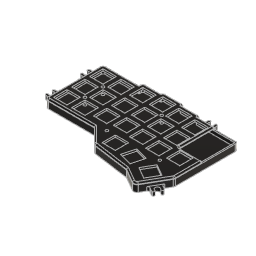
case-tenting-snap (Autodesk Fusion 360 design; units mm, degrees)
Autodesk Fusion 360 part; units mm, degrees
sketch "top_plate" plane through (0, 0, 0) normal (0, 0, 1) x (1, 0, 0)
  arc A0 (37, 57) -> (38, 58) centre (37, 58) ccw
  circle A1 centre (19, 38) radius 1.4
  circle A2 centre (76, 43) radius 1.4
  line L0 (117.5, 20.5) -> (131.5, 20.5)
  arc A3 (114, 24.5) -> (115.5, 23) centre (115.5, 24.5) ccw
  line L1 (95, 60) -> (95, 60)
  line L2 (95, 60) -> (95, 60)
  line L3 (96, 59) -> (112.5, 59)
  arc A4 (66.595, -15.7544) -> (67.4469, -16.1791) centre (67.6556, -14.6937) ccw
  line L4 (123.2697, -29.8066) -> (136.7998, -6.3468)
  arc A5 (106.318, -21.7524) -> (105.7767, -21.566) centre (105.568, -23.0514) ccw
  circle A6 centre (19, 19) radius 1.4
  line L5 (131.5, 20.5) -> (131.5, 6.5)
  line L6 (111.6878, -16.8122) -> (118.6878, -4.6878)
  line L7 (57, 62) -> (57, 62)
  arc A7 (0, 1.5) -> (1.5, 0) centre (1.5, 1.5) ccw
  line L8 (69.5, -13.5) -> (69.5, 0.5)
  line L9 (121.2203, -30.3563) -> (106.318, -21.7524)
  line L10 (118.6878, -4.6878) -> (130.8122, -11.6878)
  line L11 (58, 63) -> (75, 63)
  line L12 (38, 58) -> (38, 60)
  circle A8 centre (61, 0) radius 1.4
  line L13 (1.5, 57) -> (37, 57)
  line L14 (66.595, -15.7544) -> (51.2799, -0.4393)
  line L15 (93.5503, -0.9268) -> (107.0732, -4.5503)
  arc A9 (1.5, 57) -> (0, 55.5) centre (1.5, 55.5) ccw
  arc A10 (95, 60) -> (96, 59) centre (96, 60) ccw
  line L16 (117.5, 6.5) -> (117.5, 20.5)
  line L17 (135.5004, 23) -> (115.5, 23)
  line L18 (114, 24.5) -> (114, 57.5)
  arc A11 (121.2203, -30.3563) -> (123.2697, -29.8066) centre (121.9703, -29.0572) ccw
  arc A12 (136.7998, -6.3468) -> (137.0004, -5.5974) centre (135.5004, -5.5974) ccw
  arc A13 (76, 62) -> (75, 63) centre (75, 62) ccw
  line L19 (105.7767, -21.566) -> (67.4469, -16.1791)
  line L20 (123.8122, -23.8122) -> (111.6878, -16.8122)
  arc A14 (56, 61) -> (57, 62) centre (56, 62) ccw
  line L21 (0, 55.5) -> (0, 1.5)
  arc A15 (58, 63) -> (57, 62) centre (58, 62) ccw
  circle A16 centre (116, 1) radius 1.4
  arc A17 (39, 61) -> (38, 60) centre (39, 60) ccw
  line L22 (76, 62) -> (76, 62)
  line L23 (57, 62) -> (57, 62)
  line L24 (107.0732, -4.5503) -> (103.4497, -18.0732)
  line L25 (103.4497, -18.0732) -> (89.9268, -14.4497)
  line L26 (137.0004, 21.5) -> (137.0004, -5.5974)
  arc A18 (76, 62) -> (77, 61) centre (77, 62) ccw
  line L27 (89.9268, -14.4497) -> (93.5503, -0.9268)
  line L28 (76, 62) -> (76, 62)
  line L29 (1.5, 0) -> (50.2193, 0)
  line L30 (2.5, 40.5) -> (16.5, 40.5)
  line L31 (16.5, 40.5) -> (16.5, 54.5)
  line L32 (2.5, 54.5) -> (2.5, 40.5)
  line L33 (21.5, 2.5) -> (35.5, 2.5)
  line L34 (16.5, 35.5) -> (2.5, 35.5)
  line L35 (35.5, 2.5) -> (35.5, 16.5)
  line L36 (35.5, 21.5) -> (35.5, 35.5)
  line L37 (21.5, 16.5) -> (21.5, 2.5)
  line L38 (16.5, 54.5) -> (2.5, 54.5)
  line L39 (16.5, 21.5) -> (16.5, 35.5)
  line L40 (35.5, 16.5) -> (21.5, 16.5)
  line L41 (2.5, 35.5) -> (2.5, 21.5)
  line L42 (21.5, 21.5) -> (35.5, 21.5)
  line L43 (35.5, 35.5) -> (21.5, 35.5)
  line L44 (69.5, 0.5) -> (83.5, 0.5)
  line L45 (2.5, 21.5) -> (16.5, 21.5)
  line L46 (111.5, 42.5) -> (97.5, 42.5)
  line L47 (59.5, 8.5) -> (59.5, 22.5)
  line L48 (111.5, 37.5) -> (111.5, 23.5)
  line L49 (73.5, 46.5) -> (59.5, 46.5)
  line L50 (73.5, 41.5) -> (73.5, 27.5)
  line L51 (73.5, 22.5) -> (73.5, 8.5)
  line L52 (97.5, 18.5) -> (111.5, 18.5)
  line L53 (92.5, 39.5) -> (78.5, 39.5)
  line L54 (40.5, 20.5) -> (40.5, 6.5)
  line L55 (59.5, 27.5) -> (59.5, 41.5)
  line L56 (111.5, 4.5) -> (97.5, 4.5)
  line L57 (54.5, 44.5) -> (54.5, 58.5)
  line L58 (54.5, 20.5) -> (40.5, 20.5)
  line L59 (16.5, 2.5) -> (16.5, 16.5)
  line L60 (40.5, 39.5) -> (40.5, 25.5)
  line L61 (21.5, 40.5) -> (35.5, 40.5)
  line L62 (97.5, 56.5) -> (111.5, 56.5)
  line L63 (59.5, 60.5) -> (73.5, 60.5)
  line L64 (40.5, 44.5) -> (54.5, 44.5)
  line L65 (111.5, 56.5) -> (111.5, 42.5)
  line L66 (40.5, 25.5) -> (54.5, 25.5)
  line L67 (35.5, 40.5) -> (35.5, 54.5)
  arc A19 (95, 60) -> (94, 61) centre (94, 60) ccw
  line L68 (97.5, 23.5) -> (97.5, 37.5)
  line L69 (35.5, 54.5) -> (21.5, 54.5)
  line L70 (78.5, 39.5) -> (78.5, 25.5)
  line L71 (59.5, 22.5) -> (73.5, 22.5)
  line L72 (92.5, 44.5) -> (92.5, 58.5)
  line L73 (111.5, 23.5) -> (97.5, 23.5)
  line L74 (92.5, 25.5) -> (92.5, 39.5)
  line L75 (131.5, 6.5) -> (117.5, 6.5)
  line L76 (97.5, 4.5) -> (97.5, 18.5)
  line L77 (54.5, 58.5) -> (40.5, 58.5)
  line L78 (83.5, 0.5) -> (83.5, -13.5)
  line L79 (73.5, 8.5) -> (59.5, 8.5)
  line L80 (111.5, 18.5) -> (111.5, 4.5)
  line L81 (21.5, 35.5) -> (21.5, 21.5)
  line L82 (92.5, 6.5) -> (92.5, 20.5)
  line L83 (16.5, 16.5) -> (2.5, 16.5)
  line L84 (59.5, 41.5) -> (73.5, 41.5)
  line L85 (78.5, 6.5) -> (92.5, 6.5)
  line L86 (40.5, 58.5) -> (40.5, 44.5)
  line L87 (92.5, 20.5) -> (78.5, 20.5)
  line L88 (54.5, 25.5) -> (54.5, 39.5)
  line L89 (2.5, 16.5) -> (2.5, 2.5)
  line L90 (73.5, 27.5) -> (59.5, 27.5)
  line L91 (78.5, 25.5) -> (92.5, 25.5)
  line L92 (54.5, 6.5) -> (54.5, 20.5)
  line L93 (92.5, 58.5) -> (78.5, 58.5)
  arc A20 (137.0004, 21.5) -> (135.5004, 23) centre (135.5004, 21.5) ccw
  line L94 (130.8122, -11.6878) -> (123.8122, -23.8122)
  line L95 (39, 61) -> (56, 61)
  line L96 (77, 61) -> (94, 61)
  line L97 (40.5, 6.5) -> (54.5, 6.5)
  arc A21 (114, 57.5) -> (112.5, 59) centre (112.5, 57.5) ccw
  line L98 (97.5, 42.5) -> (97.5, 56.5)
  line L99 (78.5, 44.5) -> (92.5, 44.5)
  line L100 (21.5, 54.5) -> (21.5, 40.5)
  line L101 (73.5, 60.5) -> (73.5, 46.5)
  line L102 (59.5, 46.5) -> (59.5, 60.5)
  line L103 (54.5, 39.5) -> (40.5, 39.5)
  line L104 (78.5, 58.5) -> (78.5, 44.5)
  arc A22 (51.2799, -0.4393) -> (50.2193, 0) centre (50.2193, -1.5) ccw
  line L105 (97.5, 37.5) -> (111.5, 37.5)
  line L106 (83.5, -13.5) -> (69.5, -13.5)
  line L107 (2.5, 2.5) -> (16.5, 2.5)
  line L108 (78.5, 20.5) -> (78.5, 6.5)
  line L109 (77.8284, 63) -> (94, 63)
  arc A23 (96.8284, 61) -> (94, 63) centre (94, 60) ccw
  line L110 (96.8284, 61) -> (112.5, 61)
  line L111 (139.0004, 21.5) -> (139.0004, -5.5974)
  arc A24 (138.5323, -7.346) -> (139.0004, -5.5974) centre (135.5004, -5.5974) ccw
  line L112 (125.0022, -30.8058) -> (138.5323, -7.346)
  arc A25 (120.2203, -32.0883) -> (125.0022, -30.8058) centre (121.9703, -29.0572) ccw
  line L113 (120.2203, -32.0883) -> (105.4021, -23.5331)
  line L114 (105.4021, -23.5331) -> (67.1685, -18.1597)
  arc A26 (65.1808, -17.1686) -> (67.1685, -18.1597) centre (67.6556, -14.6937) ccw
  line L115 (65.1808, -17.1686) -> (50.0122, -2)
  line L116 (1.5, -2) -> (50.0122, -2)
  arc A27 (-2, 1.5) -> (1.5, -2) centre (1.5, 1.5) ccw
  line L117 (-2, 55.5) -> (-2, 1.5)
  arc A28 (1.5, 59) -> (-2, 55.5) centre (1.5, 55.5) ccw
  line L118 (1.5, 59) -> (36, 59)
  line L119 (36, 59) -> (36, 60)
  arc A29 (39, 63) -> (36, 60) centre (39, 60) ccw
  line L120 (39, 63) -> (55.1716, 63)
  arc A30 (58, 65) -> (55.1716, 63) centre (58, 62) ccw
  line L121 (58, 65) -> (75, 65)
  arc A31 (77.8284, 63) -> (75, 65) centre (75, 62) ccw
  line L122 (114, 57.5) -> (114, 59.5)
  line L123 (135.5004, 23) -> (137.5004, 23)
  arc A32 (114, 59.5) -> (112.5, 61) centre (112.5, 59.5) ccw
  arc A33 (139.0004, 21.5) -> (137.5004, 23) centre (137.5004, 21.5) ccw
  dimension "d10" = 1.5
  dimension "d11" = 1.5
  constraint tangent A21 L122
  constraint perpendicular L110 L122
  constraint parallel L96 L109
  constraint concentric A19 A23
  constraint parallel L3 L110
  constraint parallel L26 L111
  constraint concentric A12 A24
  constraint parallel L4 L112
  constraint concentric A11 A25
  constraint parallel L9 L113
  constraint parallel L19 L114
  constraint concentric A4 A26
  constraint parallel L14 L115
  constraint parallel L29 L116
  constraint concentric A7 A27
  constraint parallel L21 L117
  constraint concentric A9 A28
  constraint parallel L13 L118
  constraint parallel L12 L119
  constraint concentric A17 A29
  constraint parallel L95 L120
  constraint concentric A15 A30
  constraint parallel L11 L121
  constraint concentric A13 A31
  constraint tangent L109 A23
  constraint tangent A29 L120
  constraint tangent L111 A24
  constraint tangent A24 L112
  constraint tangent L112 A25
  constraint tangent A25 L113
  constraint tangent L114 A26
  constraint tangent A26 L115
  constraint tangent L116 A27
  constraint tangent A27 L117
  constraint tangent L117 A28
  constraint tangent A28 L118
  constraint tangent L119 A29
  constraint tangent A30 L121
  constraint tangent L121 A31
  constraint tangent A20 L123
  constraint perpendicular L111 L123
  constraint tangent L110 A32
  constraint tangent L122 A32
  constraint tangent L123 A33
  constraint tangent L111 A33
  measures "d10" radius of A32
  measures "d11" radius of A33
extrude "Extrude4" add sketch "top_plate" along normal blind 2 makes body 1
fillet "Fillet1" radius 1.5 27 edges at (18.75, 59, 2) (-0.9749, 57.9749, 2) (-2, 28.5, 2) (-0.9749, -0.9749, 2) (25.7561, -2, 2) (57.5965, -9.5843, 2) (66.0939, -17.826, 2) (86.2853, -20.8464, 2) (112.8112, -27.8107, 2) (122.8769, -32.4378, 2) (131.7673, -19.0759, 2) (138.8814, -6.5025, 2) (139.0004, 7.9513, 2) (138.5611, 22.5607, 2) (126.5002, 23, 2) (114.4393, 23.4393, 2) (114, 42, 2) (113.5607, 60.5607, 2) (104.6642, 61, 2) (95.7321, 62.4495, 2) (85.9142, 63, 2) (76.7321, 64.4495, 2) (66.5, 65, 2) (56.2679, 64.4495, 2) (47.0858, 63, 2) (36.8787, 62.1213, 2) (36, 59.5, 2) on bodies 1
sketch "bottom_plate" plane through (0, 0, 0) normal (0, 0, 1) x (1, 0, 0) in component "case-bottom"
  circle A0 centre (19, 38) radius 1.4
  circle A1 centre (61, 0) radius 1.4
  circle A2 centre (116, 1) radius 1.4
  arc A3 (56, 61) -> (57, 62) centre (56, 62) ccw
  circle A4 centre (76, 43) radius 1.4
  line L0 (121.2203, -30.3563) -> (106.318, -21.7524)
  line L1 (76, 62) -> (76, 62)
  line L2 (57, 62) -> (57, 62)
  line L3 (105.7767, -21.566) -> (67.4469, -16.1791)
  arc A5 (121.2203, -30.3563) -> (123.2697, -29.8066) centre (121.9703, -29.0572) ccw
  arc A6 (136.7994, -6.3479) -> (137, -5.5984) centre (135.5, -5.5984) ccw
  arc A7 (106.318, -21.7524) -> (105.7767, -21.566) centre (105.568, -23.0514) ccw
  arc A8 (76, 62) -> (75, 63) centre (75, 62) ccw
  line L4 (58, 63) -> (75, 63)
  arc A9 (95, 60) -> (96, 59) centre (96, 60) ccw
  arc A10 (0, 1.5) -> (1.5, 0) centre (1.5, 1.5) ccw
  arc A11 (51.2799, -0.4393) -> (50.2193, 0) centre (50.2193, -1.5) ccw
  line L5 (123.2697, -29.8066) -> (136.7994, -6.3479)
  arc A12 (37, 57) -> (38, 58) centre (37, 58) ccw
  arc A13 (66.595, -15.7544) -> (67.4469, -16.1791) centre (67.6556, -14.6937) ccw
  line L6 (1.5, 0) -> (50.2193, 0)
  line L7 (38, 58) -> (38, 60)
  line L8 (76, 62) -> (76, 62)
  line L9 (39, 61) -> (56, 61)
  arc A14 (39, 61) -> (38, 60) centre (39, 60) ccw
  line L10 (95, 60) -> (95, 60)
  line L11 (95, 60) -> (95, 60)
  line L12 (66.595, -15.7544) -> (51.2799, -0.4393)
  line L13 (0, 55.5) -> (0, 1.5)
  line L14 (1.5, 57) -> (37, 57)
  arc A15 (1.5, 57) -> (0, 55.5) centre (1.5, 55.5) ccw
  line L15 (77, 61) -> (94, 61)
  line L16 (57, 62) -> (57, 62)
  arc A16 (58, 63) -> (57, 62) centre (58, 62) ccw
  circle A17 centre (19, 19) radius 1.4
  line L17 (137, 57.5) -> (137, -5.5984)
  arc A18 (137, 57.5) -> (135.5, 59) centre (135.5, 57.5) ccw
  arc A19 (76, 62) -> (77, 61) centre (77, 62) ccw
  line L18 (95, 60) -> (95, 60)
  arc A20 (95, 60) -> (94, 61) centre (94, 60) ccw
  line L19 (96, 59) -> (135.5, 59)
  line L20 (96.8284, 61) -> (98, 61)
  arc A21 (139, 57.5) -> (135.5, 61) centre (135.5, 57.5) ccw
  line L21 (139, 57.5) -> (139, -5.5984)
  arc A22 (138.5319, -7.3471) -> (139, -5.5984) centre (135.5, -5.5984) ccw
  line L22 (135.2589, -13.0219) -> (138.5319, -7.3471)
  arc A23 (120.2203, -32.0883) -> (125.0022, -30.8059) centre (121.9703, -29.0572) ccw
  line L23 (120.2203, -32.0883) -> (105.4021, -23.5331)
  line L24 (105.4021, -23.5331) -> (67.1685, -18.1597)
  arc A24 (65.1808, -17.1686) -> (67.1685, -18.1597) centre (67.6556, -14.6937) ccw
  line L25 (65.1808, -17.1686) -> (50.0122, -2)
  line L26 (1.5, -2) -> (50.0122, -2)
  arc A25 (-2, 1.5) -> (1.5, -2) centre (1.5, 1.5) ccw
  line L27 (-2, 40.021) -> (-2, 17)
  arc A26 (1.5, 59) -> (-2, 55.5) centre (1.5, 55.5) ccw
  line L28 (1.5, 59) -> (36, 59)
  line L29 (36, 59) -> (36, 60)
  arc A27 (39, 63) -> (36, 60) centre (39, 60) ccw
  line L30 (39, 63) -> (55.1716, 63)
  arc A28 (58, 65) -> (55.1716, 63) centre (58, 62) ccw
  line L31 (58, 65) -> (75, 65)
  arc A29 (77.8284, 63) -> (75, 65) centre (75, 62) ccw
  line L32 (77.8284, 63) -> (94, 63)
  arc A30 (96.8284, 61) -> (94, 63) centre (94, 60) ccw
  arc A31 (95.5, 60) -> (96, 59.5) centre (96, 60) ccw
  line L33 (96, 59.5) -> (135.5, 59.5)
  arc A32 (137.5, 57.5) -> (135.5, 59.5) centre (135.5, 57.5) ccw
  line L34 (137.5, 57.5) -> (137.5, -5.5984)
  arc A33 (137.2325, -6.5977) -> (137.5, -5.5984) centre (135.5, -5.5984) ccw
  line L35 (123.7028, -30.0564) -> (137.2325, -6.5977)
  arc A34 (120.9703, -30.7893) -> (123.7028, -30.0564) centre (121.9703, -29.0572) ccw
  line L36 (120.9703, -30.7893) -> (106.068, -22.1854)
  arc A35 (106.068, -22.1854) -> (105.7071, -22.0612) centre (105.568, -23.0514) ccw
  line L37 (105.7071, -22.0612) -> (67.3773, -16.6743)
  arc A36 (66.2414, -16.1079) -> (67.3773, -16.6743) centre (67.6556, -14.6937) ccw
  line L38 (66.2414, -16.1079) -> (50.9264, -0.7929)
  arc A37 (50.9264, -0.7929) -> (50.2193, -0.5) centre (50.2193, -1.5) ccw
  line L39 (1.5, -0.5) -> (50.2193, -0.5)
  arc A38 (-0.5, 1.5) -> (1.5, -0.5) centre (1.5, 1.5) ccw
  line L40 (-0.5, 55.5) -> (-0.5, 1.5)
  arc A39 (1.5, 57.5) -> (-0.5, 55.5) centre (1.5, 55.5) ccw
  line L41 (1.5, 57.5) -> (37, 57.5)
  arc A40 (37, 57.5) -> (37.5, 58) centre (37, 58) ccw
  line L42 (37.5, 58) -> (37.5, 60)
  arc A41 (39, 61.5) -> (37.5, 60) centre (39, 60) ccw
  line L43 (39, 61.5) -> (56, 61.5)
  arc A42 (56, 61.5) -> (56.5, 62) centre (56, 62) ccw
  arc A43 (58, 63.5) -> (56.5, 62) centre (58, 62) ccw
  line L44 (58, 63.5) -> (75, 63.5)
  arc A44 (76.5, 62) -> (75, 63.5) centre (75, 62) ccw
  arc A45 (76.5, 62) -> (77, 61.5) centre (77, 62) ccw
  line L45 (77, 61.5) -> (94, 61.5)
  arc A46 (95.5, 60) -> (94, 61.5) centre (94, 60) ccw
  line L46 (1.5, 57) -> (1.5, 47) construction
  line L47 (1.5, 0) -> (1.5, 10) construction
  line L48 (1.5, 47) -> (-7.1381, 47) construction
  line L49 (1.5, 10) -> (-7, 10) construction
  circle A47 centre (-7, 10) radius 5 construction
  line L50 (-7, 10) -> (-7, 15) construction
  line L51 (-7, 10) -> (-7, 5) construction
  line L52 (-7, 15) -> (-4, 15)
  line L53 (-7, 5) -> (-4, 5)
  circle A48 centre (-7, 10) radius 2.6
  arc A49 (-7, 15) -> (-9.1131, 14.5315) centre (-7, 10) ccw
  line L54 (-7, 10) -> (-7, 15) construction
  line L55 (-7, 10) -> (-9.1131, 14.5315) construction
  arc A50 (-9.1131, 5.4685) -> (-7, 5) centre (-7, 10) ccw
  line L56 (-7, 10) -> (-9.1131, 5.4685) construction
  line L57 (-7, 10) -> (-7, 5) construction
  line L58 (-9.1131, 14.5315) -> (-8.0988, 12.3564) construction
  line L59 (-9.1131, 5.4685) -> (-8.0988, 7.6436) construction
  arc A51 (-9.1131, 14.5315) -> (-8.0988, 12.3564) centre (-8.6059, 13.444) ccw
  line L60 (-8.6059, 13.444) -> (-9.1131, 14.5315) construction
  line L61 (-8.6059, 13.444) -> (-8.0988, 12.3564) construction
  arc A52 (-8.0988, 7.6436) -> (-9.1131, 5.4685) centre (-8.6059, 6.556) ccw
  line L62 (-8.6059, 6.556) -> (-8.0988, 7.6436) construction
  line L63 (-8.6059, 6.556) -> (-9.1131, 5.4685) construction
  arc A53 (-8.2429, 44.7163) -> (-9.3647, 42.5946) centre (-8.8038, 43.6555) ccw
  arc A54 (-9.1407, 51.5463) -> (-8.1264, 49.3712) centre (-8.6335, 50.4587) ccw
  line L64 (-7.0276, 47.0148) -> (-7.2777, 42.021) construction
  arc A55 (-9.3647, 42.5946) -> (-7.2777, 42.021) centre (-7.0276, 47.0148) ccw
  line L65 (-8.6335, 50.4587) -> (-8.1264, 49.3712) construction
  line L66 (-7.1381, 47) -> (-7.2777, 42.021) construction
  line L67 (-7.1381, 47) -> (-7.0276, 52.0148) construction
  line L68 (-7.0276, 47.0148) -> (-7.0276, 52.0148) construction
  line L69 (-7.0276, 47.0148) -> (-9.3647, 42.5946) construction
  circle A56 centre (-7.0276, 47.0148) radius 2.6
  line L70 (-8.6335, 50.4587) -> (-9.1407, 51.5463) construction
  arc A57 (-7.0276, 52.0148) -> (-9.1407, 51.5463) centre (-7.0276, 47.0148) ccw
  line L71 (-9.1407, 51.5463) -> (-8.1264, 49.3712) construction
  line L72 (-9.3647, 42.5946) -> (-8.2429, 44.7163) construction
  line L73 (-7.0276, 47.0148) -> (-9.1407, 51.5463) construction
  line L74 (-8.8038, 43.6555) -> (-8.2429, 44.7163) construction
  line L75 (-8.8038, 43.6555) -> (-9.3647, 42.5946) construction
  line L76 (-7.0276, 52.0148) -> (-4, 52.0148)
  line L77 (-7.2777, 42.021) -> (-4, 42.021)
  circle A58 centre (-7.0276, 47.0148) radius 5 construction
  arc A59 (138.3204, -20.2245) -> (140.3715, -18.9783) centre (139.3459, -19.6014) ccw
  arc A60 (135.6648, -26.5557) -> (135.8729, -24.1647) centre (135.7688, -25.3602) ccw
  line L78 (136.0983, -21.5745) -> (138.8739, -17.4156) construction
  arc A61 (140.3715, -18.9783) -> (138.8739, -17.4156) centre (136.0983, -21.5745) ccw
  line L79 (135.7688, -25.3602) -> (135.8729, -24.1647) construction
  line L80 (136.6619, -21.0487) -> (138.8739, -17.4156) construction
  line L81 (136.6619, -21.0487) -> (133.6003, -25.9057) construction
  line L82 (136.0983, -21.5745) -> (133.6003, -25.9057) construction
  line L83 (136.0983, -21.5745) -> (140.3715, -18.9783) construction
  circle A62 centre (136.0983, -21.5745) radius 2.6
  line L84 (135.7688, -25.3602) -> (135.6648, -26.5557) construction
  arc A63 (133.6003, -25.9057) -> (135.6648, -26.5557) centre (136.0983, -21.5745) ccw
  line L85 (135.6648, -26.5557) -> (135.8729, -24.1647) construction
  line L86 (140.3715, -18.9783) -> (138.3204, -20.2245) construction
  line L87 (136.0983, -21.5745) -> (135.6648, -26.5557) construction
  line L88 (139.3459, -19.6014) -> (138.3204, -20.2245) construction
  line L89 (139.3459, -19.6014) -> (140.3715, -18.9783) construction
  line L90 (133.6003, -25.9057) -> (131.0015, -24.4069)
  line L91 (138.8739, -17.4156) -> (135.9922, -15.7537)
  circle A64 centre (136.0983, -21.5745) radius 5 construction
  line L92 (131.767, -19.0765) -> (136.0983, -21.5745) construction
  arc A65 (102.6436, 67.0988) -> (100.4685, 68.1131) centre (101.556, 67.6059) ccw
  arc A66 (109.5315, 68.1131) -> (107.3564, 67.0988) centre (108.444, 67.6059) ccw
  line L93 (105, 66) -> (100, 66) construction
  arc A67 (100.4685, 68.1131) -> (100, 66) centre (105, 66) ccw
  line L94 (108.444, 67.6059) -> (107.3564, 67.0988) construction
  line L95 (102.6302, 62.9627) -> (100, 66) construction
  line L96 (102.6302, 62.9627) -> (110, 66) construction
  line L97 (105, 66) -> (110, 66) construction
  line L98 (105, 66) -> (100.4685, 68.1131) construction
  circle A68 centre (105, 66) radius 2.6
  line L99 (108.444, 67.6059) -> (109.5315, 68.1131) construction
  arc A69 (110, 66) -> (109.5315, 68.1131) centre (105, 66) ccw
  line L100 (109.5315, 68.1131) -> (107.3564, 67.0988) construction
  line L101 (100.4685, 68.1131) -> (102.6436, 67.0988) construction
  line L102 (105, 66) -> (109.5315, 68.1131) construction
  line L103 (101.556, 67.6059) -> (102.6436, 67.0988) construction
  line L104 (101.556, 67.6059) -> (100.4685, 68.1131) construction
  line L105 (110, 66) -> (110, 63)
  line L106 (100, 66) -> (100, 63)
  circle A70 centre (105, 66) radius 5 construction
  line L107 (105, 61) -> (105, 66) construction
  arc A71 (-4, 15) -> (-2, 17) centre (-4, 17) ccw
  line L108 (-2, 3) -> (-2, 1.5)
  arc A72 (-2, 3) -> (-4, 5) centre (-4, 3) ccw
  arc A73 (-2, 40.021) -> (-4, 42.021) centre (-4, 40.021) ccw
  line L109 (-2, 54.0148) -> (-2, 55.5)
  arc A74 (-4, 52.0148) -> (-2, 54.0148) centre (-4, 54.0148) ccw
  arc A75 (98, 61) -> (100, 63) centre (98, 63) ccw
  line L110 (112, 61) -> (135.5, 61)
  arc A76 (110, 63) -> (112, 61) centre (112, 63) ccw
  arc A77 (135.2589, -13.0219) -> (135.9922, -15.7537) centre (136.9914, -14.0211) ccw
  line L111 (125.0022, -30.8059) -> (128.2698, -25.1402)
  arc A78 (131.0015, -24.4069) -> (128.2698, -25.1402) centre (130.0023, -26.1394) ccw
  line L112 (135.2589, -13.0219) -> (128.2698, -25.1402)
  line L113 (112, 61) -> (98, 61)
  line L114 (-2, 54.0148) -> (-2, 40.021)
  line L115 (-2, 17) -> (-2, 3)
  dimension "d24" = -0.5
  dimension "d27" = 10
  dimension "d28" = 10
  dimension "d35" = 10
  dimension "d36" = 5.2
  dimension "d37" = 25
  dimension "d38" = 25
  dimension "d39" = 180
  dimension "d40" = 180
  dimension "d41" = 10
  dimension "d42" = 10
  dimension "d45" = 10
  dimension "d46" = 5.2
  dimension "d47" = 25
  dimension "d48" = 25
  dimension "d49" = 180
  dimension "d50" = 180
  dimension "d51" = 10
  dimension "d52" = 5.2
  dimension "d53" = 25
  dimension "d54" = 25
  dimension "d55" = 180
  dimension "d56" = 180
  dimension "d57" = 5
  dimension "d58" = 10
  dimension "d59" = 5.2
  dimension "d60" = 25
  dimension "d61" = 25
  dimension "d62" = 180
  dimension "d63" = 180
  dimension "d64" = 5
  dimension "d65" = 9
  dimension "d70" = 2
  dimension "d71" = 2
  dimension "d72" = 2
  dimension "d73" = 2
  dimension "d74" = 2
  dimension "d75" = 2
  dimension "d76" = 2
  dimension "d77" = 2
  constraint perpendicular L14 L46
  constraint perpendicular L6 L47
  constraint perpendicular L46 L48
  constraint perpendicular L27 L49
  constraint tangent L27 A47
  constraint coincident A47 L50.end
  constraint perpendicular L49 L50
  constraint coincident A47 L51.end
  constraint perpendicular L49 L51
  constraint tangent A47 L52
  constraint perpendicular L27 L52
  constraint perpendicular L27 L53
  constraint concentric A47 A48
  constraint coincident L49.end A47.centre
  constraint coincident A48 L58.end
  constraint coincident L55 L58.end
  constraint coincident A48 L59.end
  constraint coincident L56 L59.end
  constraint midpoint L58 A51.centre
  constraint coincident L67.end A58
  constraint coincident L64.end A58
  constraint tangent L76 A58
  constraint concentric A56 A58
  constraint coincident L64.start A55.centre
  constraint coincident A54.end A56
  constraint coincident A54.end L73
  constraint coincident A53.start A56
  constraint coincident A53.start L69
  constraint midpoint A54.centre L71
  constraint coincident L81.end A64
  constraint coincident L78.end A64
  constraint tangent L90 A64
  constraint concentric A62 A64
  constraint coincident L78.start A61.centre
  constraint coincident A60.end A62
  constraint coincident A60.end L87
  constraint coincident A59.start A62
  constraint coincident A59.start L83
  constraint midpoint A60.centre L85
  constraint perpendicular L22 L92
  constraint perpendicular L22 L91
  constraint coincident L96.end A70
  constraint coincident L93.end A70
  constraint tangent L105 A70
  constraint concentric A68 A70
  constraint coincident L93.start A67.centre
  constraint coincident A66.end A68
  constraint coincident A66.end L102
  constraint coincident A65.start A68
  constraint coincident A65.start L98
  constraint midpoint A66.centre L100
  constraint coincident L20 L107.start
  constraint perpendicular L20 L107
  constraint vertical L106
  constraint vertical L105
  constraint horizontal L93
  constraint horizontal L76
  constraint horizontal L77
  constraint perpendicular L22 L90
  constraint parallel L19 L20
  constraint concentric A18 A21
  constraint parallel L17 L21
  constraint concentric A6 A22
  constraint parallel L5 L22
  constraint concentric A5 A23
  constraint parallel L0 L23
  constraint parallel L3 L24
  constraint concentric A13 A24
  constraint parallel L12 L25
  constraint parallel L6 L26
  constraint concentric A10 A25
  constraint parallel L13 L27
  constraint concentric A15 A26
  constraint parallel L14 L28
  constraint parallel L7 L29
  constraint concentric A14 A27
  constraint parallel L9 L30
  constraint concentric A16 A28
  constraint parallel L4 L31
  constraint concentric A8 A29
  constraint parallel L15 L32
  constraint concentric A20 A30
  constraint tangent A21 L21
  constraint tangent L20 A21
  constraint tangent A25 L27
  constraint tangent L21 A22
  constraint tangent A22 L22
  constraint tangent A23 L23
  constraint tangent L32 A30
  constraint tangent L24 A24
  constraint tangent A24 L25
  constraint tangent L26 A25
  constraint coincident A25.start L27
  constraint tangent L52 A71
  constraint tangent L27 A71
  constraint tangent A25 L108
  constraint tangent L53 A72
  constraint tangent L108 A72
  constraint coincident A26.end L27
  constraint tangent L77 A73
  constraint tangent L27 A73
  constraint tangent A26 L109
  constraint tangent L76 A74
  constraint tangent L109 A74
  constraint coincident A21.end L20
  constraint tangent L20 A75
  constraint tangent L106 A75
  constraint tangent A21 L110
  constraint tangent L110 A76
  constraint tangent L105 A76
  constraint coincident L22 L92.start
  constraint tangent L91 A77
  constraint tangent L22 A77
  constraint perpendicular L90 L111
  constraint tangent L90 A78
  constraint tangent L111 A78
  constraint tangent A78 L112
  constraint tangent A75 L113
  constraint tangent A72 L115
  measures "d27" distance of L14.start L46.end
  measures "d28" distance of A10.end L47.end
  measures "d35" diameter of A47
  measures "d36" diameter of A48
  measures "d37" angle of L54 L55
  measures "d38" angle of L56 L57
  measures "d39" angle of L60 L61
  measures "d40" angle of L62 L63
  measures "d41" distance of L14.start L46.end
  measures "d42" distance of A10.end L47.end
  measures "d45" diameter of A58
  measures "d46" diameter of A56
  measures "d47" angle of L68 L73
  measures "d48" angle of L64 L69
  measures "d49" angle of L65 L70
  measures "d50" angle of L74 L75
  measures "d51" diameter of A64
  measures "d52" diameter of A62
  measures "d53" angle of L82 L87
  measures "d54" angle of L78 L83
  measures "d55" angle of L79 L84
  measures "d56" angle of L88 L89
  measures "d57" distance of L92.start L78.start
  measures "d58" diameter of A70
  measures "d59" diameter of A68
  measures "d60" angle of L97 L102
  measures "d61" angle of L93 L98
  measures "d62" angle of L94 L99
  measures "d63" angle of L103 L104
  measures "d64" distance of L107.start L93.start
  measures "d65" horizontal distance of A31.end L107.start
  measures "d70" radius of A71
  measures "d71" radius of A72
  measures "d72" radius of A73
  measures "d73" radius of A74
  measures "d74" radius of A75
  measures "d75" radius of A76
  measures "d76" radius of A77
  measures "d77" radius of A78
extrude "Extrude4'" add sketch "bottom_plate" along normal blind 5 separate body contours L20 A21 L21 A22 L22 A23 L23 L24 A24 L25 L26 A25 L27 A26 L28 L29 A27 L30 A28 L31 A29 L32 A30 L108 L109 L110 L111 L112 L113 L114 L115 makes body 2 in component "case-bottom"
extrude "Extrude3" add sketch "bottom_plate" against normal blind 2 contours A3 L0 L3 A5 A6 A7 A8 L4 A9 A10 A11 L5 A12 A13 L6 L7 L9 A14 L12 L13 L14 A15 L15 A16 L17 A18 A19 A20 L19 | L20 A21 L21 A22 L22 A23 L23 L24 A24 L25 L26 A25 L27 A26 L28 L29 A27 L30 A28 L31 A29 L32 A30 L108 L109 L110 L111 L112 L113 L114 L115 | A31 L33 A32 L34 A33 L35 A34 L36 A35 L37 A36 L38 A37 L39 A38 L40 A39 L41 A40 L42 A41 L43 A42 A43 L44 A44 A45 L45 A46 bodies 2 in component "case-bottom"
move_body "Move1" bodies 1 to x (1, 0, 0) y (0, 1, 0) z (0, 0, 1) at (0, 0, 7)
move_body "Move2" bodies 1 to x (1, 0, 0) y (0, 1, 0) z (0, 0, 1) at (0, 0, -2)
sketch "Sketch5" plane through (0, 0, 5) normal (0, 0, 1) x (-1, 0, 0)
  arc A0 (-139, -57.5) -> (-135.5, -61) centre (-135.5, -57.5) ccw
  line L0 (-135.5, -61) -> (-96.8284, -61)
  arc A1 (-96.8284, -61) -> (-94, -63) centre (-94, -60) ccw
  line L1 (-94, -63) -> (-77.8284, -63)
  arc A2 (-77.8284, -63) -> (-75, -65) centre (-75, -62) ccw
  line L2 (-75, -65) -> (-58, -65)
  arc A3 (-58, -65) -> (-55.1716, -63) centre (-58, -62) ccw
  line L3 (-55.1716, -63) -> (-39, -63)
  arc A4 (-39, -63) -> (-36, -60) centre (-39, -60) ccw
  line L4 (-36, -60) -> (-36, -59)
  line L5 (-36, -59) -> (-1.5, -59)
  arc A5 (-1.5, -59) -> (2, -55.5) centre (-1.5, -55.5) ccw
  line L6 (2, -40.021) -> (2, -1.5)
  arc A6 (2, -1.5) -> (-1.5, 2) centre (-1.5, -1.5) ccw
  line L7 (-1.5, 2) -> (-50.0122, 2)
  line L8 (-50.0122, 2) -> (-65.1808, 17.1686)
  arc A7 (-65.1808, 17.1686) -> (-67.1685, 18.1597) centre (-67.6556, 14.6937) ccw
  line L9 (-67.1685, 18.1597) -> (-105.4021, 23.5331)
  line L10 (-105.4021, 23.5331) -> (-120.2203, 32.0883)
  arc A8 (-120.2203, 32.0883) -> (-125.0022, 30.8059) centre (-121.9703, 29.0572) ccw
  line L11 (-125.0022, 30.8059) -> (-138.5319, 7.3471)
  arc A9 (-138.5319, 7.3471) -> (-139, 5.5984) centre (-135.5, 5.5984) ccw
  line L12 (-139, 5.5984) -> (-139, -57.5)
  line L13 (-137, -57.5) -> (-137, -61)
  line L14 (-114, -59) -> (-135.5, -59)
  line L15 (-114, -59) -> (-114, -61)
  line L16 (-114, -61) -> (-137, -61)
  arc A10 (-95.5, -60) -> (-96, -59.5) centre (-96, -60) ccw
  line L17 (-96, -59.5) -> (-135.5, -59.5)
  arc A11 (-137.5, -57.5) -> (-135.5, -59.5) centre (-135.5, -57.5) ccw
  line L18 (-137.5, -57.5) -> (-137.5, 5.5984)
  arc A12 (-137.2325, 6.5977) -> (-137.5, 5.5984) centre (-135.5, 5.5984) ccw
  line L19 (-137.2325, 6.5977) -> (-123.7028, 30.0564)
  arc A13 (-120.9703, 30.7893) -> (-123.7028, 30.0564) centre (-121.9703, 29.0572) ccw
  line L20 (-120.9703, 30.7893) -> (-106.068, 22.1854)
  arc A14 (-106.068, 22.1854) -> (-105.7071, 22.0612) centre (-105.568, 23.0514) ccw
  line L21 (-105.7071, 22.0612) -> (-67.3773, 16.6743)
  arc A15 (-66.2414, 16.1079) -> (-67.3773, 16.6743) centre (-67.6556, 14.6937) ccw
  line L22 (-66.2414, 16.1079) -> (-50.9264, 0.7929)
  arc A16 (-50.9264, 0.7929) -> (-50.2193, 0.5) centre (-50.2193, 1.5) ccw
  line L23 (-50.2193, 0.5) -> (-1.5, 0.5)
  arc A17 (0.5, -1.5) -> (-1.5, 0.5) centre (-1.5, -1.5) ccw
  line L24 (0.5, -1.5) -> (0.5, -55.5)
  arc A18 (-1.5, -57.5) -> (0.5, -55.5) centre (-1.5, -55.5) ccw
  line L25 (-1.5, -57.5) -> (-37, -57.5)
  arc A19 (-37, -57.5) -> (-37.5, -58) centre (-37, -58) ccw
  line L26 (-37.5, -58) -> (-37.5, -60)
  arc A20 (-39, -61.5) -> (-37.5, -60) centre (-39, -60) ccw
  line L27 (-39, -61.5) -> (-56, -61.5)
  arc A21 (-56, -61.5) -> (-56.5, -62) centre (-56, -62) ccw
  arc A22 (-58, -63.5) -> (-56.5, -62) centre (-58, -62) ccw
  line L28 (-58, -63.5) -> (-75, -63.5)
  arc A23 (-76.5, -62) -> (-75, -63.5) centre (-75, -62) ccw
  arc A24 (-76.5, -62) -> (-77, -61.5) centre (-77, -62) ccw
  line L29 (-77, -61.5) -> (-94, -61.5)
  arc A25 (-95.5, -60) -> (-94, -61.5) centre (-94, -60) ccw
  line L30 (2, -55.5) -> (2, -54.0148)
  line L31 (2, -54.0148) -> (2, -40.021)
  constraint coincident L0 L15.end
  constraint perpendicular L0 L15
  constraint perpendicular L13 L16
extrude "Extrude5" cut sketch "Sketch5" against normal blind 1 contours A0 L0 L13 L15 L16 L17 A11 | A0 L13 L16 bodies 2 in component "case-bottom"
extrude "Extrude6" add sketch "bottom_plate" along normal blind 2 contours L20 A21 L21 A22 L22 A23 L23 L24 A24 L25 L26 A25 L27 A26 L28 L29 A27 L30 A28 L31 A29 L32 A30 L108 L109 L110 L111 L112 L113 L114 L115 | A65 A66 A67 A68 A69 L105 L106 A75 A76 L113 | A59 A60 A61 A62 A63 L90 L91 A77 A78 L112 | A53 A54 A55 A56 A57 L76 L77 A73 A74 L114 | L52 L53 A48 A49 A50 A51 A52 A71 A72 L115 | A31 L33 A32 L34 A33 L35 A34 L36 A35 L37 A36 L38 A37 L39 A38 L40 A39 L41 A40 L42 A41 L43 A42 A43 L44 A44 A45 L45 A46 bodies 2 in component "case-bottom"
extrude "Extrude7" add 4 faces at (132.7549, -19.6176, 0) (-3.1281, 10.0644, 0) (-3.1351, 46.9952, 0) (104.9356, 62.1281, 0) along direction (0, 0, -1) blind 2 on bodies 2 bodies 2 in component "case-bottom"
extrude "Extrude8" cut 1 faces at (137.1667, 15.4344, 2) along direction (0, 0, -1) blind 2 on bodies 2 bodies 2 in component "case-bottom"
copy_body "Body->Comp1" bodies 1 removing the originals makes body 3 in component "case-top"
component "case-bottom" placed x (1, 0, 0) y (0, 1, 0) z (0, 0, 1) at (0, 0, 0)
component "case-top" placed x (1, 0, 0) y (0, 1, 0) z (0, 0, 1) at (0, 0, 0)
equation "d37 = snap_angle"
equation "d38 = snap_angle"
equation "snap_angle = 25 deg"
equation "d47 = snap_angle"
equation "d48 = snap_angle"
equation "d53 = snap_angle"
equation "d54 = snap_angle"
equation "d60 = snap_angle"
equation "d61 = snap_angle"
named bodies: "case-top", "case-bottom"
